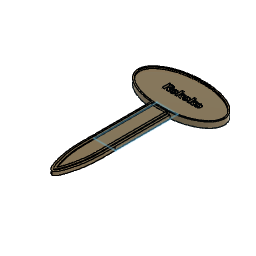
Rosen-Tafel_Rokoko v1 (Autodesk Fusion 360 design; units mm, degrees)
Autodesk Fusion 360 part; units mm, degrees
sketch "Skizze1" plane through (0, 0, 0) normal (0, 0, 1) x (1, 0, 0) in component "Tafe"
  ellipse E0 centre (0, 0) end of major axis (60, 0) minor radius 30
  line L0 (-60, 0) -> (60, 0)
  line L1 (0, -30) -> (0, 30)
  dimension "d1" = 60
  constraint coincident E0.centre origin
  constraint horizontal L0
  constraint coincident E0 L0.start
  constraint coincident E0 L0.end
  constraint coincident E0 L1.start
  constraint coincident E0 L1.end
  measures "d1" distance of E0
extrude "Extrusion1" add sketch "Skizze1" along normal blind 3 makes body 1 in component "Tafe"
sketch "Skizze2" plane through (0, 0, 3) normal (0, 0, 1) x (-1, 0, 0) in component "Tafe"
  ellipse E0 centre (0, 0) end of major axis (-60, 0) minor radius 30
  spline S0 degree 3 poles (61.9509, 0) (61.9509, 4.2635) (60.3055, 8.4828) (57.3091, 12.2636) (52.6449, 18.1488) (44.7166, 23.0684) (34.8255, 26.4973) (25.2136, 29.8294) (13.7584, 31.7256) (2.1658, 31.9316) (-9.8896, 32.1459) (-22.0459, 30.5274) (-32.3487, 27.3124) (-41.3637, 24.4992) (-48.9522, 20.4892) (-54.1681, 15.6411) (-58.1005, 11.9859) (-60.7028, 7.8251) (-61.5993, 3.4465) (-62.4053, -0.4903) (-61.7899, -4.5541) (-59.8722, -8.3093) (-56.3973, -15.1137) (-48.7697, -20.9418) (-38.5998, -25.0786) (-29.6788, -28.7075) (-18.796, -31.0188) (-7.5068, -31.7189) (4.0223, -32.434) (15.9353, -31.462) (26.4461, -28.9362) (36.7725, -26.4548) (45.7187, -22.4959) (52.0049, -17.4981) (56.4978, -13.926) (59.6597, -9.8063) (61.0885, -5.3839) (61.6588, -3.6187) (61.9509, -1.8099) (61.9509, 0) knots -3.141593 -3.141593 -3.141593 -3.141593 -2.764311 -2.764311 -2.764311 -2.177028 -2.177028 -2.177028 -1.606323 -1.606323 -1.606323 -1.012833 -1.012833 -1.012833 -0.49353 -0.49353 -0.49353 -0.102016 -0.102016 -0.102016 0.249996 0.249996 0.249996 0.887852 0.887852 0.887852 1.447382 1.447382 1.447382 2.018805 2.018805 2.018805 2.580199 2.580199 2.580199 2.981436 2.981436 2.981436 3.141593 3.141593 3.141593 3.141593
  dimension "d4" = 1.9509
extrude "Extrusion2" add sketch "Skizze2" along normal blind 2 and the other way blind 2 bodies 1 in component "Tafe"
sketch "Skizze3" plane through (0, 0, 0) normal (0, 0, 1) x (1, 0, 0) in component "Tafe"
extrude "Extrusion3" add 1 faces at (23.0091, -28.1834, 1) along direction (0, 0, -1) blind 1 on bodies 1 bodies 1 in component "Tafe"
sketch "Skizze1 (2)" plane through (0, 0, 0) normal (0, 0, 1) x (1, 0, 0) in component "Ständer"
extrude "Extrusion4" add 2 faces at (23.0091, -28.1834, 0) (8.4972, -9.7981, 0) along direction (0, 0, -1) blind 3 on bodies 1 bodies 1 in component "Tafe"
sketch "Skizze2 (2)" plane through (0, 0, -3) normal (0, 0, -1) x (1, 0, 0) in component "Ständer"
  spline S0 degree 3 poles (-61.9509, 0) (-61.9509, -1.8099) (-61.6588, -3.6187) (-61.0885, -5.3839) (-59.6597, -9.8063) (-56.4978, -13.926) (-52.0049, -17.4981) (-45.7187, -22.4959) (-36.7725, -26.4548) (-26.4461, -28.9362) (-15.9353, -31.462) (-4.0223, -32.434) (7.5068, -31.7189) (18.796, -31.0188) (29.6788, -28.7075) (38.5998, -25.0786) (48.7697, -20.9418) (56.3973, -15.1137) (59.8722, -8.3093) (61.7899, -4.5541) (62.4053, -0.4903) (61.5993, 3.4465) (60.7028, 7.8251) (58.1005, 11.9859) (54.1681, 15.6411) (48.9522, 20.4892) (41.3637, 24.4992) (32.3487, 27.3124) (22.0459, 30.5274) (9.8896, 32.1459) (-2.1658, 31.9316) (-13.7584, 31.7256) (-25.2136, 29.8294) (-34.8255, 26.4973) (-44.7166, 23.0684) (-52.6449, 18.1488) (-57.3091, 12.2636) (-60.3055, 8.4828) (-61.9509, 4.2635) (-61.9509, 0) knots -3.141593 -3.141593 -3.141593 -3.141593 -2.981436 -2.981436 -2.981436 -2.580199 -2.580199 -2.580199 -2.018805 -2.018805 -2.018805 -1.447382 -1.447382 -1.447382 -0.887852 -0.887852 -0.887852 -0.249996 -0.249996 -0.249996 0.102016 0.102016 0.102016 0.49353 0.49353 0.49353 1.012833 1.012833 1.012833 1.606323 1.606323 1.606323 2.177028 2.177028 2.177028 2.764311 2.764311 2.764311 3.141593 3.141593 3.141593 3.141593
  line L0 (15, 20) -> (-15, 20)
  line L1 (-15, 20) -> (-15, 110)
  line L2 (-15, 110) -> (15, 110)
  line L3 (15, 110) -> (15, 20)
  constraint horizontal L0
  constraint vertical L1
  constraint horizontal L2
  constraint vertical L3
extrude "Extrusion1'" add sketch "Skizze2 (2)" against normal blind 5 separate body contours S0 L0 L1 L3 picked at (1.6815, 23.9477) makes body 2 in component "Ständer"
extrude "Extrusion2'" add sketch "Skizze2 (2)" against normal blind 5 contours S0 L1 L2 L3 bodies 2 in component "Ständer"
sketch "Skizze3 (2)" plane through (0, 0, 2) normal (0, 0, 1) x (-1, 0, 0) in component "Ständer"
  line L0 (15, 20) -> (15, 110)
  line L1 (15, 110) -> (-15, 110)
  line L2 (-15, 110) -> (-15, 20)
  line L3 (-15, 20) -> (15, 20)
  spline S0 degree 5 poles (15, 110) (15.0176, 110.8619) (15.0503, 112.5708) (15.0915, 115.0899) (15.1309, 118.3598) (15.1537, 122.2987) (15.1484, 126.0898) (15.1122, 129.7366) (15.0406, 133.2467) (14.9275, 136.6331) (14.7639, 139.9163) (14.5397, 143.1226) (14.2439, 146.2818) (13.867, 149.4242) (13.4012, 152.5784) (12.8426, 155.769) (12.1915, 159.0132) (11.4507, 162.3163) (10.6251, 165.6668) (9.72, 169.0317) (8.7408, 172.3517) (7.6913, 175.5347) (6.574, 178.4677) (5.3908, 181.0335) (4.1426, 183.1253) (2.8302, 184.6621) (1.7296, 185.4171) (0.8758, 185.7125) (0.294, 185.7893) (0, 185.7977) knots 0 0 0 0 0 0 0.04 0.08 0.12 0.16 0.2 0.24 0.28 0.32 0.36 0.4 0.44 0.48 0.52 0.56 0.6 0.64 0.68 0.72 0.76 0.8 0.84 0.88 0.92 0.96 1 1 1 1 1 1
  line L4 (0, -2.5) -> (0, -20)
  spline S1 degree 5 poles (-15, 110) (-15.0176, 110.8619) (-15.0503, 112.5708) (-15.0915, 115.0899) (-15.1309, 118.3598) (-15.1537, 122.2987) (-15.1484, 126.0898) (-15.1122, 129.7366) (-15.0406, 133.2467) (-14.9275, 136.6331) (-14.7639, 139.9163) (-14.5397, 143.1226) (-14.2439, 146.2818) (-13.867, 149.4242) (-13.4012, 152.5784) (-12.8426, 155.769) (-12.1915, 159.0132) (-11.4507, 162.3163) (-10.6251, 165.6668) (-9.72, 169.0317) (-8.7408, 172.3517) (-7.6913, 175.5347) (-6.574, 178.4677) (-5.3908, 181.0335) (-4.1426, 183.1253) (-2.8302, 184.6621) (-1.7296, 185.4171) (-0.8758, 185.7125) (-0.294, 185.7893) (0, 185.7977) knots 0 0 0 0 0 0 0.04 0.08 0.12 0.16 0.2 0.24 0.28 0.32 0.36 0.4 0.44 0.48 0.52 0.56 0.6 0.64 0.68 0.72 0.76 0.8 0.84 0.88 0.92 0.96 1 1 1 1 1 1
  line L5 (14.8117, 100.8471) -> (15.1883, 119.1529)
  line L6 (6.7737, 185.6047) -> (-6.7737, 185.9906)
  line L7 (-14.8117, 100.8471) -> (-15.1883, 119.1529)
  line L8 (-6.7737, 185.6047) -> (6.7737, 185.9906)
  point P0 (15, 134.2579)
  point P1 (13.5579, 151.4378)
  point P2 (9.54, 169.5876)
  point P3 (3.9981, 183.1652)
  point P4 (-15, 134.2579)
  point P5 (-13.5579, 151.4378)
  point P6 (-9.54, 169.5876)
  point P7 (-3.9981, 183.1652)
  constraint coincident L0.end L1.start
  constraint midpoint L0.end L5
  constraint midpoint S0.end L6
  constraint symmetric L0.end L4 L1.end
  constraint symmetric P0 L4 P4
  constraint symmetric P1 L4 P5
  constraint symmetric P2 L4 P6
  constraint symmetric P3 L4 P7
  constraint symmetric S0.end L4 S1.end
  constraint symmetric L4 L5.start L7.start
  constraint symmetric L4 L5.end L7.end
  constraint symmetric L4 L6.start L8.start
  constraint symmetric L4 L6.end L8.end
extrude "Extrusion3'" add sketch "Skizze3 (2)" against normal blind 5 contours L1 S0 S1 bodies 2 in component "Ständer"
sketch "Skizze4" plane through (0, 0, 2) normal (0, 0, 1) x (-1, 0, 0) in component "Ständer"
  line L0 (15, 20) -> (15, 110)
  spline S0 degree 5 poles (15, 110) (15.0176, 110.8619) (15.0503, 112.5708) (15.0915, 115.0899) (15.1309, 118.3598) (15.1537, 122.2987) (15.1484, 126.0898) (15.1122, 129.7366) (15.0406, 133.2467) (14.9275, 136.6331) (14.7639, 139.9163) (14.5397, 143.1226) (14.2439, 146.2818) (13.867, 149.4242) (13.4012, 152.5784) (12.8426, 155.769) (12.1915, 159.0132) (11.4507, 162.3163) (10.6251, 165.6668) (9.72, 169.0317) (8.7408, 172.3517) (7.6913, 175.5347) (6.574, 178.4677) (5.3908, 181.0335) (4.1426, 183.1253) (2.8302, 184.6621) (1.7296, 185.4171) (0.8758, 185.7125) (0.294, 185.7893) (0, 185.7977) knots 0 0 0 0 0 0 0.04 0.08 0.12 0.16 0.2 0.24 0.28 0.32 0.36 0.4 0.44 0.48 0.52 0.56 0.6 0.64 0.68 0.72 0.76 0.8 0.84 0.88 0.92 0.96 1 1 1 1 1 1
  spline S1 degree 5 poles (-15, 110) (-15.0176, 110.8619) (-15.0503, 112.5708) (-15.0915, 115.0899) (-15.1309, 118.3598) (-15.1537, 122.2987) (-15.1484, 126.0898) (-15.1122, 129.7366) (-15.0406, 133.2467) (-14.9275, 136.6331) (-14.7639, 139.9163) (-14.5397, 143.1226) (-14.2439, 146.2818) (-13.867, 149.4242) (-13.4012, 152.5784) (-12.8426, 155.769) (-12.1915, 159.0132) (-11.4507, 162.3163) (-10.6251, 165.6668) (-9.72, 169.0317) (-8.7408, 172.3517) (-7.6913, 175.5347) (-6.574, 178.4677) (-5.3908, 181.0335) (-4.1426, 183.1253) (-2.8302, 184.6621) (-1.7296, 185.4171) (-0.8758, 185.7125) (-0.294, 185.7893) (0, 185.7977) knots 0 0 0 0 0 0 0.04 0.08 0.12 0.16 0.2 0.24 0.28 0.32 0.36 0.4 0.44 0.48 0.52 0.56 0.6 0.64 0.68 0.72 0.76 0.8 0.84 0.88 0.92 0.96 1 1 1 1 1 1
  line L1 (-15, 110) -> (-15, 20)
  line L2 (-15, 20) -> (15, 20)
  spline S2 degree 3 poles (-11.9777, 110.0309) (-11.9779, 110.0412) (-11.9781, 110.0515) (-11.9783, 110.0618) (-12.1467, 118.2962) (-12.1876, 125.6884) (-12.0304, 132.2915) (-11.8915, 138.1249) (-11.5879, 143.3276) (-10.915, 148.5264) (-10.4464, 152.1476) (-9.7926, 155.8041) (-8.949, 159.6156) (-8.1726, 163.1233) (-7.2391, 166.7794) (-6.1929, 170.2595) (-5.0109, 174.1918) (-3.6533, 177.8638) (-2.3593, 180.1318) (-1.7058, 181.2772) (-1.0734, 182.0403) (-0.6357, 182.4064) (-0.297, 182.6897) (-0.1153, 182.7456) (0, 182.7673) knots -0.000287 -0.000287 -0.000287 -0.000287 0 0 0 0.23016 0.23016 0.23016 0.433487 0.433487 0.433487 0.575116 0.575116 0.575116 0.705456 0.705456 0.705456 0.852728 0.852728 0.852728 0.927106 0.927106 0.927106 0.984664 0.984664 0.984664 0.984664
  spline S3 degree 3 poles (11.9777, 110.0309) (11.9779, 110.0412) (11.9781, 110.0515) (11.9783, 110.0618) (12.1467, 118.2962) (12.1876, 125.6884) (12.0304, 132.2915) (11.8915, 138.1249) (11.5879, 143.3276) (10.915, 148.5264) (10.4464, 152.1476) (9.7926, 155.8041) (8.949, 159.6156) (8.1726, 163.1233) (7.2391, 166.7794) (6.1929, 170.2595) (5.0109, 174.1918) (3.6533, 177.8638) (2.3593, 180.1318) (1.7058, 181.2772) (1.0734, 182.0403) (0.6357, 182.4064) (0.297, 182.6897) (0.1153, 182.7456) (0, 182.7673) knots -0.000287 -0.000287 -0.000287 -0.000287 0 0 0 0.23016 0.23016 0.23016 0.433487 0.433487 0.433487 0.575116 0.575116 0.575116 0.705456 0.705456 0.705456 0.852728 0.852728 0.852728 0.927106 0.927106 0.927106 0.984664 0.984664 0.984664 0.984664
  line L3 (11.9777, 23.0223) -> (11.9777, 110.0309)
  line L4 (-11.9777, 23.0223) -> (11.9777, 23.0223)
  line L5 (-11.9777, 110.0309) -> (-11.9777, 23.0223)
  spline S4 degree 3 poles (-9, 110.0613) (-9.0004, 110.0818) (-9.0008, 110.1022) (-9.0013, 110.1226) (-9.1708, 118.4153) (-9.2103, 125.8461) (-9.0484, 132.4316) (-8.9146, 137.8751) (-8.6346, 142.7164) (-8.0427, 147.5055) (-7.6174, 150.9474) (-7.0241, 154.4041) (-6.2475, 158.0272) (-5.5493, 161.2843) (-4.705, 164.6878) (-3.7598, 167.9778) (-2.8347, 171.1978) (-1.801, 174.2968) (-0.8034, 176.5706) (-0.5276, 177.1992) (-0.2561, 177.763) (0, 178.2439) knots -0.000569 -0.000569 -0.000569 -0.000569 0 0 0 0.232641 0.232641 0.232641 0.424939 0.424939 0.424939 0.56314 0.56314 0.56314 0.687378 0.687378 0.687378 0.80897 0.80897 0.80897 0.842587 0.842587 0.842587 0.842587
  spline S5 degree 3 poles (9, 110.0613) (9.0004, 110.0818) (9.0008, 110.1022) (9.0013, 110.1226) (9.1708, 118.4153) (9.2103, 125.8461) (9.0484, 132.4316) (8.9146, 137.8751) (8.6346, 142.7164) (8.0427, 147.5055) (7.6174, 150.9474) (7.0241, 154.4041) (6.2475, 158.0272) (5.5493, 161.2843) (4.705, 164.6878) (3.7598, 167.9778) (2.8347, 171.1978) (1.801, 174.2968) (0.8034, 176.5706) (0.5276, 177.1992) (0.2561, 177.763) (0, 178.2439) knots -0.000569 -0.000569 -0.000569 -0.000569 0 0 0 0.232641 0.232641 0.232641 0.424939 0.424939 0.424939 0.56314 0.56314 0.56314 0.687378 0.687378 0.687378 0.80897 0.80897 0.80897 0.842587 0.842587 0.842587 0.842587
  line L6 (9, 26) -> (9, 110.0613)
  line L7 (-9, 26) -> (9, 26)
  line L8 (-9, 110.0613) -> (-9, 26)
  dimension "d19" = -3.0223
  dimension "d20" = -6
extrude "Extrusion4'" add sketch "Skizze4" along normal blind 1 contours S2 S3 L3 L4 L5 bodies 2 in component "Ständer"
combine "Kombinieren1" operation add target body 1 tool bodies 2 in component "Tafe"
sketch "Skizze1 (3)" plane through (0, 0, 3) normal (0, 0, 1) x (-1, 0, 0)
  ellipse E0 centre (0, 0) end of major axis (-60, 0) minor radius 30
  line L0 (19.3194, -7.1042) -> (17.9551, -7.1042)
  spline S0 degree 2 poles (17.9551, -7.1042) (17.1616, -7.1042) (16.532, -6.8345) knots 0 0 0 1 1 1
  spline S1 degree 2 poles (16.532, -6.8345) (15.9023, -6.5648) (15.4638, -6.1106) knots 0 0 0 1 1 1
  spline S2 degree 2 poles (15.4638, -6.1106) (15.0252, -5.6563) (14.7918, -5.0531) knots 0 0 0 1 1 1
  spline S3 degree 2 poles (14.7918, -5.0531) (14.5584, -4.4499) (14.5584, -3.7828) knots 0 0 0 1 1 1
  spline S4 degree 2 poles (14.5584, -3.7828) (14.5584, -2.8035) (14.8555, -2.1648) knots 0 0 0 1 1 1
  spline S5 degree 2 poles (14.8555, -2.1648) (15.1526, -1.526) (15.5064, -1.1572) knots 0 0 0 1 1 1
  spline S6 degree 2 poles (15.5064, -1.1572) (15.9307, -0.717) (16.4541, -0.4901) knots 0 0 0 1 1 1
  line L1 (16.4541, -0.4901) -> (14.0041, 3.8816)
  line L2 (14.0041, 3.8816) -> (17.4727, 3.8816)
  line L3 (17.4727, 3.8816) -> (19.3194, 0.1581)
  line L4 (19.3194, 0.1581) -> (19.3194, -2.1868)
  spline S7 degree 2 poles (19.3194, -2.1868) (19.0209, -2.2011) (18.7296, -2.2579) knots 0 0 0 1 1 1
  spline S8 degree 2 poles (18.7296, -2.2579) (18.4383, -2.3148) (18.2038, -2.464) knots 0 0 0 1 1 1
  spline S9 degree 2 poles (18.2038, -2.464) (17.9693, -2.6132) (17.8271, -2.8761) knots 0 0 0 1 1 1
  spline S10 degree 2 poles (17.8271, -2.8761) (17.685, -3.139) (17.685, -3.5654) knots 0 0 0 1 1 1
  spline S11 degree 2 poles (17.685, -3.5654) (17.685, -4.1907) (18.0901, -4.4892) knots 0 0 0 1 1 1
  spline S12 degree 2 poles (18.0901, -4.4892) (18.4951, -4.7876) (19.0778, -4.7876) knots 0 0 0 1 1 1
  line L5 (19.0778, -4.7876) -> (19.3194, -4.7876)
  line L6 (19.3194, -4.7876) -> (19.3194, -7.1042)
  line L7 (20.57, 3.8816) -> (23.6682, 3.8816)
  line L8 (23.6682, 3.8816) -> (23.6682, -7.1042)
  line L9 (23.6682, -7.1042) -> (20.57, -7.1042)
  line L10 (20.57, -7.1042) -> (20.57, 3.8816)
  spline S13 degree 2 poles (10.8917, -1.121) (11.2328, -0.9504) (11.446, -0.6164) knots 0 0 0 1 1 1
  spline S14 degree 2 poles (11.446, -0.6164) (11.6592, -0.2825) (11.6592, 0.1297) knots 0 0 0 1 1 1
  spline S15 degree 2 poles (11.6592, 0.1297) (11.6592, 0.5134) (11.446, 0.8474) knots 0 0 0 1 1 1
  spline S16 degree 2 poles (11.446, 0.8474) (11.2328, 1.1814) (10.8917, 1.3519) knots 0 0 0 1 1 1
  line L11 (10.8917, 1.3519) -> (10.8917, 4.0237)
  spline S17 degree 2 poles (10.8917, 4.0237) (11.7018, 3.9243) (12.3556, 3.5832) knots 0 0 0 1 1 1
  spline S18 degree 2 poles (12.3556, 3.5832) (13.0093, 3.2421) (13.457, 2.7234) knots 0 0 0 1 1 1
  spline S19 degree 2 poles (13.457, 2.7234) (13.9047, 2.2046) (14.1463, 1.5367) knots 0 0 0 1 1 1
  spline S20 degree 2 poles (14.1463, 1.5367) (14.3879, 0.8687) (14.3879, 0.1297) knots 0 0 0 1 1 1
  spline S21 degree 2 poles (14.3879, 0.1297) (14.3879, -0.6235) (14.1463, -1.2986) knots 0 0 0 1 1 1
  spline S22 degree 2 poles (14.1463, -1.2986) (13.9047, -1.9737) (13.4499, -2.4924) knots 0 0 0 1 1 1
  spline S23 degree 2 poles (13.4499, -2.4924) (12.9951, -3.0111) (12.3485, -3.3522) knots 0 0 0 1 1 1
  spline S24 degree 2 poles (12.3485, -3.3522) (11.7018, -3.6933) (10.8917, -3.7928) knots 0 0 0 1 1 1
  line L12 (10.8917, -3.7928) -> (10.8917, -1.121)
  spline S25 degree 2 poles (8.8879, 0.1297) (8.8879, -0.2825) (9.0939, -0.6164) knots 0 0 0 1 1 1
  spline S26 degree 2 poles (9.0939, -0.6164) (9.3, -0.9504) (9.6553, -1.121) knots 0 0 0 1 1 1
  line L13 (9.6553, -1.121) -> (9.6553, -3.7928)
  spline S27 degree 2 poles (9.6553, -3.7928) (8.8452, -3.6933) (8.1986, -3.3451) knots 0 0 0 1 1 1
  spline S28 degree 2 poles (8.1986, -3.3451) (7.5519, -2.9969) (7.0972, -2.4711) knots 0 0 0 1 1 1
  spline S29 degree 2 poles (7.0972, -2.4711) (6.6424, -1.9452) (6.4008, -1.2773) knots 0 0 0 1 1 1
  spline S30 degree 2 poles (6.4008, -1.2773) (6.1592, -0.6093) (6.1592, 0.1297) knots 0 0 0 1 1 1
  spline S31 degree 2 poles (6.1592, 0.1297) (6.1592, 0.8545) (6.3937, 1.5225) knots 0 0 0 1 1 1
  spline S32 degree 2 poles (6.3937, 1.5225) (6.6282, 2.1904) (7.0759, 2.7091) knots 0 0 0 1 1 1
  spline S33 degree 2 poles (7.0759, 2.7091) (7.5235, 3.2279) (8.1773, 3.5761) knots 0 0 0 1 1 1
  spline S34 degree 2 poles (8.1773, 3.5761) (8.831, 3.9243) (9.6553, 4.0237) knots 0 0 0 1 1 1
  line L14 (9.6553, 4.0237) -> (9.6553, 1.3519)
  spline S35 degree 2 poles (9.6553, 1.3519) (9.3142, 1.1814) (9.101, 0.8474) knots 0 0 0 1 1 1
  spline S36 degree 2 poles (9.101, 0.8474) (8.8879, 0.5134) (8.8879, 0.1297) knots 0 0 0 1 1 1
  line L15 (1.2561, -2.5706) -> (0.5739, -3.6649)
  line L16 (0.5739, -3.6649) -> (-2.9648, -3.6649)
  line L17 (-2.9648, -3.6649) -> (-0.3783, -0.0124)
  line L18 (-0.3783, -0.0124) -> (-3.2633, 3.8816)
  line L19 (-3.2633, 3.8816) -> (0.2186, 3.8816)
  line L20 (0.2186, 3.8816) -> (1.2561, 2.3467)
  line L21 (1.2561, 2.3467) -> (1.2561, -2.5706)
  line L22 (2.4641, 3.8816) -> (5.2923, 3.8816)
  line L23 (5.2923, 3.8816) -> (5.2923, -7.1184)
  line L24 (5.2923, -7.1184) -> (2.4641, -7.1184)
  line L25 (2.4641, -7.1184) -> (2.4641, 3.8816)
  spline S37 degree 2 poles (-6.7026, -1.121) (-6.3615, -0.9504) (-6.1483, -0.6164) knots 0 0 0 1 1 1
  spline S38 degree 2 poles (-6.1483, -0.6164) (-5.9351, -0.2825) (-5.9351, 0.1297) knots 0 0 0 1 1 1
  spline S39 degree 2 poles (-5.9351, 0.1297) (-5.9351, 0.5134) (-6.1483, 0.8474) knots 0 0 0 1 1 1
  spline S40 degree 2 poles (-6.1483, 0.8474) (-6.3615, 1.1814) (-6.7026, 1.3519) knots 0 0 0 1 1 1
  line L26 (-6.7026, 1.3519) -> (-6.7026, 4.0237)
  spline S41 degree 2 poles (-6.7026, 4.0237) (-5.8925, 3.9243) (-5.2388, 3.5832) knots 0 0 0 1 1 1
  spline S42 degree 2 poles (-5.2388, 3.5832) (-4.585, 3.2421) (-4.1373, 2.7234) knots 0 0 0 1 1 1
  spline S43 degree 2 poles (-4.1373, 2.7234) (-3.6897, 2.2046) (-3.4481, 1.5367) knots 0 0 0 1 1 1
  spline S44 degree 2 poles (-3.4481, 1.5367) (-3.2065, 0.8687) (-3.2065, 0.1297) knots 0 0 0 1 1 1
  spline S45 degree 2 poles (-3.2065, 0.1297) (-3.2065, -0.6235) (-3.4481, -1.2986) knots 0 0 0 1 1 1
  spline S46 degree 2 poles (-3.4481, -1.2986) (-3.6897, -1.9737) (-4.1444, -2.4924) knots 0 0 0 1 1 1
  spline S47 degree 2 poles (-4.1444, -2.4924) (-4.5992, -3.0111) (-5.2459, -3.3522) knots 0 0 0 1 1 1
  spline S48 degree 2 poles (-5.2459, -3.3522) (-5.8925, -3.6933) (-6.7026, -3.7928) knots 0 0 0 1 1 1
  line L27 (-6.7026, -3.7928) -> (-6.7026, -1.121)
  spline S49 degree 2 poles (-8.7065, 0.1297) (-8.7065, -0.2825) (-8.5004, -0.6164) knots 0 0 0 1 1 1
  spline S50 degree 2 poles (-8.5004, -0.6164) (-8.2943, -0.9504) (-7.939, -1.121) knots 0 0 0 1 1 1
  line L28 (-7.939, -1.121) -> (-7.939, -3.7928)
  spline S51 degree 2 poles (-7.939, -3.7928) (-8.7491, -3.6933) (-9.3957, -3.3451) knots 0 0 0 1 1 1
  spline S52 degree 2 poles (-9.3957, -3.3451) (-10.0424, -2.9969) (-10.4972, -2.4711) knots 0 0 0 1 1 1
  spline S53 degree 2 poles (-10.4972, -2.4711) (-10.9519, -1.9452) (-11.1935, -1.2773) knots 0 0 0 1 1 1
  spline S54 degree 2 poles (-11.1935, -1.2773) (-11.4351, -0.6093) (-11.4351, 0.1297) knots 0 0 0 1 1 1
  spline S55 degree 2 poles (-11.4351, 0.1297) (-11.4351, 0.8545) (-11.2006, 1.5225) knots 0 0 0 1 1 1
  spline S56 degree 2 poles (-11.2006, 1.5225) (-10.9661, 2.1904) (-10.5185, 2.7091) knots 0 0 0 1 1 1
  spline S57 degree 2 poles (-10.5185, 2.7091) (-10.0708, 3.2279) (-9.417, 3.5761) knots 0 0 0 1 1 1
  spline S58 degree 2 poles (-9.417, 3.5761) (-8.7633, 3.9243) (-7.939, 4.0237) knots 0 0 0 1 1 1
  line L29 (-7.939, 4.0237) -> (-7.939, 1.3519)
  spline S59 degree 2 poles (-7.939, 1.3519) (-8.2801, 1.1814) (-8.4933, 0.8474) knots 0 0 0 1 1 1
  spline S60 degree 2 poles (-8.4933, 0.8474) (-8.7065, 0.5134) (-8.7065, 0.1297) knots 0 0 0 1 1 1
  line L30 (-16.3382, -2.5706) -> (-17.0204, -3.6649)
  line L31 (-17.0204, -3.6649) -> (-20.5592, -3.6649)
  line L32 (-20.5592, -3.6649) -> (-17.9726, -0.0124)
  line L33 (-17.9726, -0.0124) -> (-20.8576, 3.8816)
  line L34 (-20.8576, 3.8816) -> (-17.3757, 3.8816)
  line L35 (-17.3757, 3.8816) -> (-16.3382, 2.3467)
  line L36 (-16.3382, 2.3467) -> (-16.3382, -2.5706)
  line L37 (-15.1302, 3.8816) -> (-12.3021, 3.8816)
  line L38 (-12.3021, 3.8816) -> (-12.3021, -7.1184)
  line L39 (-12.3021, -7.1184) -> (-15.1302, -7.1184)
  line L40 (-15.1302, -7.1184) -> (-15.1302, 3.8816)
  spline S61 degree 2 poles (-24.2969, -1.121) (-23.9558, -0.9504) (-23.7426, -0.6164) knots 0 0 0 1 1 1
  spline S62 degree 2 poles (-23.7426, -0.6164) (-23.5294, -0.2825) (-23.5294, 0.1297) knots 0 0 0 1 1 1
  spline S63 degree 2 poles (-23.5294, 0.1297) (-23.5294, 0.5134) (-23.7426, 0.8474) knots 0 0 0 1 1 1
  spline S64 degree 2 poles (-23.7426, 0.8474) (-23.9558, 1.1814) (-24.2969, 1.3519) knots 0 0 0 1 1 1
  line L41 (-24.2969, 1.3519) -> (-24.2969, 4.0237)
  spline S65 degree 2 poles (-24.2969, 4.0237) (-23.4868, 3.9243) (-22.8331, 3.5832) knots 0 0 0 1 1 1
  spline S66 degree 2 poles (-22.8331, 3.5832) (-22.1793, 3.2421) (-21.7316, 2.7234) knots 0 0 0 1 1 1
  spline S67 degree 2 poles (-21.7316, 2.7234) (-21.284, 2.2046) (-21.0424, 1.5367) knots 0 0 0 1 1 1
  spline S68 degree 2 poles (-21.0424, 1.5367) (-20.8008, 0.8687) (-20.8008, 0.1297) knots 0 0 0 1 1 1
  spline S69 degree 2 poles (-20.8008, 0.1297) (-20.8008, -0.6235) (-21.0424, -1.2986) knots 0 0 0 1 1 1
  spline S70 degree 2 poles (-21.0424, -1.2986) (-21.284, -1.9737) (-21.7387, -2.4924) knots 0 0 0 1 1 1
  spline S71 degree 2 poles (-21.7387, -2.4924) (-22.1935, -3.0111) (-22.8402, -3.3522) knots 0 0 0 1 1 1
  spline S72 degree 2 poles (-22.8402, -3.3522) (-23.4868, -3.6933) (-24.2969, -3.7928) knots 0 0 0 1 1 1
  line L42 (-24.2969, -3.7928) -> (-24.2969, -1.121)
  spline S73 degree 2 poles (-26.3008, 0.1297) (-26.3008, -0.2825) (-26.0947, -0.6164) knots 0 0 0 1 1 1
  spline S74 degree 2 poles (-26.0947, -0.6164) (-25.8886, -0.9504) (-25.5333, -1.121) knots 0 0 0 1 1 1
  line L43 (-25.5333, -1.121) -> (-25.5333, -3.7928)
  spline S75 degree 2 poles (-25.5333, -3.7928) (-26.3434, -3.6933) (-26.99, -3.3451) knots 0 0 0 1 1 1
  spline S76 degree 2 poles (-26.99, -3.3451) (-27.6367, -2.9969) (-28.0915, -2.4711) knots 0 0 0 1 1 1
  spline S77 degree 2 poles (-28.0915, -2.4711) (-28.5462, -1.9452) (-28.7878, -1.2773) knots 0 0 0 1 1 1
  spline S78 degree 2 poles (-28.7878, -1.2773) (-29.0294, -0.6093) (-29.0294, 0.1297) knots 0 0 0 1 1 1
  spline S79 degree 2 poles (-29.0294, 0.1297) (-29.0294, 0.8545) (-28.7949, 1.5225) knots 0 0 0 1 1 1
  spline S80 degree 2 poles (-28.7949, 1.5225) (-28.5605, 2.1904) (-28.1128, 2.7091) knots 0 0 0 1 1 1
  spline S81 degree 2 poles (-28.1128, 2.7091) (-27.6651, 3.2279) (-27.0114, 3.5761) knots 0 0 0 1 1 1
  spline S82 degree 2 poles (-27.0114, 3.5761) (-26.3576, 3.9243) (-25.5333, 4.0237) knots 0 0 0 1 1 1
  line L44 (-25.5333, 4.0237) -> (-25.5333, 1.3519)
  spline S83 degree 2 poles (-25.5333, 1.3519) (-25.8744, 1.1814) (-26.0876, 0.8474) knots 0 0 0 1 1 1
  spline S84 degree 2 poles (-26.0876, 0.8474) (-26.3008, 0.5134) (-26.3008, 0.1297) knots 0 0 0 1 1 1
extrude "Extrusion5" cut sketch "Skizze1 (3)" against normal blind 33 contours L0 S0 S1 S2 S3 S4 S5 S6 L1 L2 L3 L4 S7 S8 S9 S10 S11 S12 L5 L6 | L7 L8 L9 L10 | S13 S14 S15 S16 L11 S17 S18 S19 S20 S21 S22 S23 S24 L12 | S25 S26 L13 S27 S28 S29 S30 S31 S32 S33 S34 L14 S35 S36 | L15 L16 L17 L18 L19 L20 L21 | L22 L23 L24 L25 | S37 S38 S39 S40 L26 S41 S42 S43 S44 S45 S46 S47 S48 L27 | S49 S50 L28 S51 S52 S53 S54 S55 S56 S57 S58 L29 S59 S60 | L30 L31 L32 L33 L34 L35 L36 | L37 L38 L39 L40 | S61 S62 S63 S64 L41 S65 S66 S67 S68 S69 S70 S71 S72 L42 | S73 S74 L43 S75 S76 S77 S78 S79 S80 S81 S82 L44 S83 S84 bodies 1 in component "Tafe"
component "Tafe" placed x (1, 0, 0) y (0, 1, 0) z (0, 0, 1) at (0, 0, 0)
component "Ständer" placed x (1, 0, 0) y (0, 1, 0) z (0, 0, 1) at (0, 0, 0)
named bodies: "Grundplatte"
